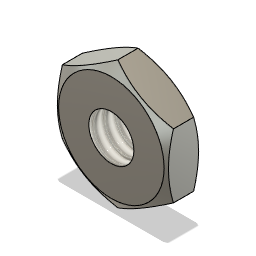
Sofle_Chico_v3.5.x_FDM v8 (Autodesk Fusion 360 archive; units mm, degrees)
design "Hexagon Nut BS 4183 - M2 Steel 6 Plain"
description: Hexagon Nut BS 4183 - M2
Autodesk Fusion 360 part; units mm, degrees
sketch "Sketch1" plane through (0, 0, 0) normal (0, 1, 0) x (1, 0, 0)
  line L0 (0, 0) -> (0, -1.2)
  line L1 (-1, 0) -> (-1.9, 0)
  line L2 (-1.9, 0) -> (-2.31, -0.2367)
  line L3 (-2.31, -0.2367) -> (-2.31, -0.9633)
  line L4 (-2.31, -0.9633) -> (-1.9, -1.2)
  line L5 (-1.9, -1.2) -> (-1, -1.2)
  line L6 (-1, -1.2) -> (-1, 0)
  line L7 (-1, 0) -> (0, 0) construction
  line L8 (-1, -1.2) -> (0, -1.2) construction
  dimension "d121" = 2
  dimension "d122" = 30
  dimension "d123" = 30
  dimension "d125" = 3.8
  dimension "d126" = 1.2
  dimension "d127" = 3.8
  dimension "d128" = 4.62
  constraint vertical L0
  constraint coincident L0 L8.end
  constraint coincident L7.end L0
  constraint horizontal L1
  constraint perpendicular L1 L3
  constraint perpendicular L3 L5
  constraint perpendicular L5 L6
  constraint coincident L0.start L1
  constraint coincident L0.start L7.end
  constraint perpendicular L0 L8
  measures "d122" angle of L1 L2
  measures "d123" angle of L4 L5
  measures "d126" distance of L1.start L5.end
revolve "Revolve1" add sketch "Sketch1" angle 360 about axis through (0, 0, 0) along (0, 0, 1)
sketch "Sketch8" plane through (0, 0, 1.2) normal (0, 0, 1) x (1, 0, 0)
  line L0 (0, 0) -> (-4, 0) construction
  line L1 (-2, -1.1559) -> (-2, 1.1559)
  circle A0 centre (0, 0) radius 1
  circle A1 centre (0, 0) radius 2.31
  dimension "d114" = 2
  constraint horizontal L0
  constraint perpendicular L0 L1
  constraint midpoint L0 L1
  constraint coincident L0.start A0.centre
  constraint coincident L1.end A1
  measures "d114" distance of L0.start L1
extrude "Extrude5" cut sketch "Sketch8" against normal blind 1.2 contours L1 A1 picked at (-2.05, 0.2815)
pattern_circular "C-Pattern2" count 6 over 360 about axis through (0, 0, 1.75) along (0, 0, 1) of "Extrude5"
thread "Thread3" "ISO Metric profile 2.0 M2x0.4 6H" major diameter 2.074 minor diameter 1.623 pitch 0.4 angle 60 resizes the face on face at (-0.995, 0.0996, 0.8)
equation "adsk_nheig = 1.20 mm"
equation "adsk_maxdia = 4.62 mm"
equation "adsk_nomdia = 2.00 mm"
equation "d89 = -adsk_nheig"
equation "adsk_waflat = 4.00 mm"
equation "d114 = adsk_waflat / 2"
equation "adsk_chamang1 = 30 deg"
equation "adsk_chamang2 = 30 deg"
equation "d121 = adsk_nomdia"
equation "d122 = adsk_chamang1"
equation "d123 = adsk_chamang2"
equation "d125 = adsk_waflat * 0.95"
equation "d126 = adsk_nheig"
equation "d127 = adsk_waflat * 0.95"
equation "d128 = adsk_maxdia"
equation "d147 = adsk_nheig"
